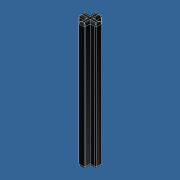
# Autodesk Inventor part: 3705
Saved by Autodesk Inventor 2011 SP2 (Build 150553200, 553)
## iProperties
Created: 2011-11-29
Part Number: 3705
Cost Center: 0 kg
Material: Steel
Document SubType Name: Modeling
Designer: PMe
Authority: 0 mm^3
Stock Number: =<Filenr>_<Document number>
Mass: 2.9567 g
Surface Area: 5.62668 cm^2
Volume: 0.37665 cm^3
Density: 7.85 g/cm^3
Company: Allseas Engineering BV
Subject: =<Title><TITLE 1_2> <TITLE 2_2>
Author: PMe
Act. Code: DW000
SaveDate: 2011-07-28
SaveTime: 18:32
FileName: Standard
TotalMass: 0 kg
TotalVolume: 0 mm^3
Autodesk Inventor part; units mm, degrees
ref_plane "YZ Plane" through (0, 0, 0) normal (1, 0, 0) x (0, 1, 0)
ref_plane "XZ Plane" through (0, 0, 0) normal (0, 1, 0) x (-1, 0, 0)
ref_plane "XY Plane" through (0, 0, 0) normal (0, 0, 1) x (1, 0, 0)
sketch "Sketch1" plane through (0, 0, 0) normal (0, 0, 1) x (1, 0, 0)
  circle A0 centre (0, 0) radius 2.3
  line L0 (-2.1564, 0.8) -> (-0.8, 0.8)
  line L1 (-0.8, 0.8) -> (-0.8, 2.1564)
  line L2 (0.8, 2.1564) -> (0.8, 0.8)
  line L3 (0.8, 0.8) -> (2.1564, 0.8)
  line L4 (2.1564, -0.8) -> (0.8, -0.8)
  line L5 (0.8, -0.8) -> (0.8, -2.1564)
  line L6 (-0.8, -2.1564) -> (-0.8, -0.8)
  line L7 (-0.8, -0.8) -> (-2.1564, -0.8)
  dimension "d0" = 4.6
  dimension "d1" = 1.6
  constraints: 16 end point, 4 perpendicular, 3 equal length, 3 parallel, 2 horizontal alignment, 2 vertical alignment, 1 coincident, 1 horizontal, 10 other
  measures "d1" distance between parallel lines of L2 L1
extrude "Extrusion1" add sketch "Sketch1" along normal mid plane 32 contours A0 L4 L5 L6 L7 L0 L1 L2 L3
fillet "Fillet1" radius 0.5 24 edges at (0, 2.3, 16) (0.8, 1.4782, 16) (1.4782, 0.8, 16) (2.3, 0, 16) (1.4782, -0.8, 16) (0.8, -1.4782, 16) (0, -2.3, 16) (-0.8, -1.4782, 16) (-1.4782, -0.8, 16) (-2.3, 0, 16) (-1.4782, 0.8, 16) (-0.8, 1.4782, 16) (0, 2.3, -16) (-2.3, 0, -16) (0, -2.3, -16) (2.3, 0, -16) (1.4782, 0.8, -16) (0.8, 1.4782, -16) (-0.8, 1.4782, -16) (-1.4782, 0.8, -16) (-1.4782, -0.8, -16) (-0.8, -1.4782, -16) (0.8, -1.4782, -16) (1.4782, -0.8, -16)
fillet "Fillet2" radius 0.2 24 edges at (0.8, 2.1564, 0) (0.6467, 2.047, 15.8603) (0.6467, 2.047, -15.8603) (-0.8, 2.1564, 0) (-0.6467, 2.047, 15.8603) (-0.6467, 2.047, -15.8603) (-2.1564, 0.8, 0) (-2.047, 0.6467, -15.8603) (-2.047, 0.6467, 15.8603) (-2.1564, -0.8, 0) (-2.047, -0.6467, 15.8603) (-2.047, -0.6467, -15.8603) (-0.8, -2.1564, 0) (-0.6467, -2.047, 15.8603) (-0.6467, -2.047, -15.8603) (0.8, -2.1564, 0) (0.6467, -2.047, 15.8603) (0.6467, -2.047, -15.8603) (2.1564, -0.8, 0) (2.047, -0.6467, 15.8603) (2.047, -0.6467, -15.8603) (2.1564, 0.8, 0) (2.047, 0.6467, 15.8603) (2.047, 0.6467, -15.8603)
body "Solid1"
